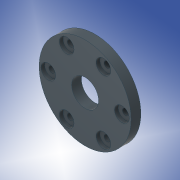
# Autodesk Inventor part: BA007
Saved by Autodesk Inventor 2017 SP1 (Build 210196100, 196)
## iProperties
Created: 2017-06-15
Part Number: BA007
Material: ABS Plastic
Document SubType Name: Modeling
Designer: zallen
Density: 1.06 g/cm^3
Appearance: CR Dark Blue
Author: zallen
Autodesk Inventor part; units mm, degrees
ref_plane "YZ Plane" through (0, 0, 0) normal (1, 0, 0) x (0, 1, 0)
ref_plane "XZ Plane" through (0, 0, 0) normal (0, 1, 0) x (-1, 0, 0)
ref_plane "XY Plane" through (0, 0, 0) normal (0, 0, 1) x (1, 0, 0)
sketch "Sketch8" plane through (0, 0, 0) normal (0, 0, 1) x (1, 0, 0)
  circle A0 centre (30, 0) radius 2.5
  circle A1 centre (15, 25.9808) radius 2.5
  circle A2 centre (-15, 25.9808) radius 2.5
  circle A3 centre (-30, 0) radius 2.5
  circle A4 centre (-15, -25.9808) radius 2.5
  circle A5 centre (15, -25.9808) radius 2.5
  circle A6 centre (0, 0) radius 37.5
  circle A7 centre (0, 0) radius 11
  dimension "d53" = 5
  dimension "d54" = 30
  dimension "d57" = 360
  dimension "d59" = 75
  dimension "d60" = 22
  constraints: 8 centre point, 2 coincident, 1 horizontal alignment, 13 other
  measures "d53" diameter of A0
  measures "d54" distance of A0.centre point (0, 0)
  measures "d59" diameter of A6
  measures "d60" diameter of A7
extrude "Extrusion8" add sketch "Sketch8" along normal blind 8
sketch "Sketch9" plane through (0, 0, 8) normal (0, 0, 1) x (1, 0, 0)
  circle A0 centre (-15, 25.9808) radius 2.5 projected
  circle A1 centre (15, 25.9808) radius 2.5 projected
  circle A2 centre (30, 0) radius 2.5 projected
  circle A3 centre (15, -25.9808) radius 2.5 projected
  circle A4 centre (-15, -25.9808) radius 2.5 projected
  circle A5 centre (-30, 0) radius 2.5 projected
  circle A6 centre (-15, 25.9808) radius 2.5 projected
  circle A7 centre (-15, 25.9808) radius 6
  circle A8 centre (-30, 0) radius 6
  circle A9 centre (-15, -25.9808) radius 6
  circle A10 centre (15, -25.9808) radius 6
  circle A11 centre (30, 0) radius 6
  circle A12 centre (15, 25.9808) radius 6
  point P0 (0, 0)
  dimension "d63" = 12
  dimension "d66" = 360
  constraints: 6 centre point, 1 coincident, 19 other
  measures "d63" diameter of A7
extrude "Extrusion9" cut sketch "Sketch9" against normal blind 3 contours A0 | A1 | A2 | A3 | A4 | A5 | A7 | A8 | A9 | A10 | A11 | A12
body "Solid2"
